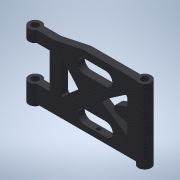
# Autodesk Inventor part: Left_upper_part
Saved by Autodesk Inventor 2020 (Build 240168000, 168)
## iProperties
Created: 2015-12-03
Part Number: Left_upper_part
Material: Acero, suave
Document SubType Name: Modeling
Designer: MIGUEL ANGEL
Density: 7.85 g/cm^3
Appearance: Hierro - Fundido
Author: MIGUEL ANGEL
Autodesk Inventor part; units mm, degrees
ref_plane "YZ Plane" through (0, 0, 0) normal (1, 0, 0) x (0, 1, 0)
ref_plane "XZ Plane" through (0, 0, 0) normal (0, 1, 0) x (-1, 0, 0)
sketch "Boceto2" plane through (0, 0, 0) normal (0, 0, 1) x (1, 0, 0)
  circle A0 centre (-16.7491, 0.2224) radius 9
  circle A1 centre (138.5611, 0.2224) radius 9
  line L0 (-9.2658, 5.2224) -> (131.0778, 5.2224)
  line L1 (131.0778, -4.7776) -> (-9.2658, -4.7776)
  circle A2 centre (138.5611, 0.2224) radius 5
  circle A3 centre (-16.7491, 0.2224) radius 5
  point P0 (0, 0)
  dimension "d2" = 18
  dimension "d3" = 10
  dimension "d4" = 10
  constraints: 4 centre point, 4 end point, 4 point on circle, 2 coincident, 2 equal radius, 2 horizontal
  measures "d2" diameter of A0
  measures "d3" diameter of A3
  measures "d4" distance between parallel lines of L1 L0
extrude "Extrusión1" add sketch "Boceto2" along normal blind 100 contours A0 L0 A1 L1
ref_plane "Plano de trabajo1" through (0, 0, 50) normal (0, 0, -1) x (-1, 0, 0)
sketch "Boceto3" plane through (0, 0, 50) normal (0, 0, -1) x (-1, 0, 0)
  circle A0 centre (-138.5611, 0.2224) radius 9 projected
  circle A1 centre (16.7491, 0.2224) radius 9 projected
  circle A2 centre (-138.5611, 0.2224) radius 5 projected
  circle A3 centre (16.7491, 0.2224) radius 5 projected
  point P0 (0, 0)
extrude "Extrusión2" add sketch "Boceto3" along normal mid plane 105
sketch "Boceto4" plane through (0, 0, 0) normal (0, 1, 0) x (-1, 0, 0)
  line L0 (25.7491, 102.5) -> (25.7491, -2.5) projected
  line L1 (9.2658, 0) -> (-131.0778, 0) projected
  line L2 (9.2658, 100) -> (-131.0778, 100) projected
  line L3 (-147.5611, 102.5) -> (-147.5611, -2.5) projected
  line L4 (25.7491, 9) -> (-14.9531, 9)
  line L5 (-14.9531, 9) -> (-57.3933, 0)
  line L6 (9.2658, 0) -> (-131.0778, 0) projected
  line L7 (-57.3933, 100) -> (-14.9531, 91)
  line L8 (-14.9531, 91) -> (25.7491, 91)
  line L9 (25.7491, 75) -> (-8.8807, 75)
  line L10 (-8.8807, 75) -> (-8.8807, 25)
  line L11 (-8.8807, 25) -> (25.7491, 25)
  line L12 (-24.9356, 70.614) -> (-24.9356, 29.386)
  line L13 (-83.4051, 51.7146) -> (-115.5189, 73.8108)
  line L14 (-118.6526, 72.1632) -> (-118.6526, 61.0832)
  line L15 (-118.6526, 39.8101) -> (-118.6526, 28.73)
  line L16 (-115.5457, 27.0642) -> (-83.4319, 48.4011)
  line L17 (-28.4456, 71.9255) -> (-48.8564, 48.4239)
  line L18 (-28.247, 27.8759) -> (-48.6578, 45.6025)
  line L19 (-57.9307, 80) -> (-88.0143, 80) construction
  line L20 (-57.9307, 89.5575) -> (-88.0143, 89.5575)
  line L21 (-88.0143, 70.4425) -> (-57.9307, 70.4425)
  arc A0 (-57.9307, 70.4425) -> (-57.9307, 89.5575) centre (-57.9307, 80) ccw
  arc A1 (-88.0143, 89.5575) -> (-88.0143, 70.4425) centre (-88.0143, 80) ccw
  line L22 (-57.9307, 18.0061) -> (-88.508, 18.0061) construction
  line L23 (-57.9307, 27.6984) -> (-88.508, 27.6984)
  line L24 (-88.508, 8.3137) -> (-57.9307, 8.3137)
  arc A2 (-57.9307, 8.3137) -> (-57.9307, 27.6984) centre (-57.9307, 18.0061) ccw
  arc A3 (-88.508, 27.6984) -> (-88.508, 8.3137) centre (-88.508, 18.0061) ccw
  line L25 (-118.6526, 61.0832) -> (-103.6526, 55.6402)
  arc A4 (-105.6651, 44.0001) -> (-103.6526, 55.6402) centre (-105.6992, 50) ccw
  line L26 (-105.6651, 44.0001) -> (-117.037, 41.7728)
  arc A5 (-115.5189, 73.8108) -> (-118.6526, 72.1632) centre (-116.6526, 72.1632) ccw
  arc A6 (-83.4319, 48.4011) -> (-83.4051, 51.7146) centre (-84.5388, 50.0669) ccw
  arc A7 (-118.6526, 28.73) -> (-115.5457, 27.0642) centre (-116.6526, 28.73) ccw
  arc A8 (-117.037, 41.7728) -> (-118.6526, 39.8101) centre (-116.6526, 39.8101) ccw
  arc A9 (-28.247, 27.8759) -> (-24.9356, 29.386) centre (-26.9356, 29.386) ccw
  arc A10 (-24.9356, 70.614) -> (-28.4456, 71.9255) centre (-26.9356, 70.614) ccw
  arc A11 (-48.8564, 48.4239) -> (-48.6578, 45.6025) centre (-47.3464, 47.1125) ccw
  line L27 (25.7491, 100) -> (25.7491, 91)
  line L28 (7.7491, 102.5) -> (7.7491, -2.5) projected
  line L29 (-57.3933, 100) -> (7.7491, 100)
  line L30 (7.7491, 102.5) -> (25.7491, 102.5)
  line L31 (25.7491, 102.5) -> (7.7491, 102.5) projected
  point P0 (0, 0)
  point P1 (-24.9356, 75.967)
  point P2 (-24.9356, 25)
  point P3 (-80.9683, 50.038)
  point P4 (-118.6526, 75.967)
  point P5 (-118.6526, 41.4563)
  point P6 (-118.6526, 25)
  point P7 (-8.8807, 50)
  point P8 (25.7491, 50)
  point P9 (-24.9356, 50)
  point P10 (-50.1679, 46.9139)
  point P11 (-72.9725, 80)
  point P12 (-73.2193, 18.0061)
  point P13 (-147.5611, 50)
  dimension "d11" = 50
  dimension "d12" = 16
  dimension "d14" = 16
  dimension "d26" = 2
  dimension "d27" = 2
  dimension "d28" = 6
  dimension "d29" = 15
  constraints: 54 end point, 27 point on line, 24 point on circle, 23 tangent, 12 centre point, 6 midpoint, 6 perpendicular, 5 equal radius, 5 horizontal alignment, 3 collinear, 3 parallel, 2 horizontal, 2 vertical alignment, 1 vertical
  measures "d11" distance between parallel lines of L11 L9
  measures "d12" distance between parallel lines of L9 L8
  measures "d14" distance between parallel lines of L11 L4
  measures "d26" radius of A5
  measures "d27" radius of A9
  measures "d28" radius of A4
  measures "d29" horizontal distance of L14.end L25.end
extrude "Extrusión4" cut sketch "Boceto4" along normal through all both and the other way through all contours L0 L8 L28 L30 | L28 L8 L7 L2 | L0 L11 L28 L9 | L28 L11 L10 L9 | L12 A9 L18 A11 L17 A10 | A6 L16 A7 L15 A8 L26 A4 L25 L14 A5 L13 | A0 L21 A1 L20 | A2 L24 A3 L23
sketch "Boceto5" plane through (57.9307, 5.2224, 8.3137) normal (0, 0, 1) x (1, 0, 0)
  line L0 (0, 0) -> (30.5774, 0) projected
  line L1 (0, -10) -> (0, 0) projected
  line L2 (30.5774, -10) -> (0, -10) projected
  line L3 (30.5774, -10) -> (30.5774, 0) projected
  circle A0 centre (15.2887, -5) radius 3
  line L4 (0, 0) -> (30.5774, 0) projected
  line L5 (0, -10) -> (0, 0) projected
  point P0 (-57.9307, -5.2224)
  point P1 (15.2887, 0)
  point P2 (0, -5)
  dimension "d32" = 6
  constraints: 2 midpoint, 1 centre point, 1 horizontal alignment, 1 vertical alignment
  measures "d32" diameter of A0
extrude "Extrusión5" cut sketch "Boceto5" against normal through all contours A0
